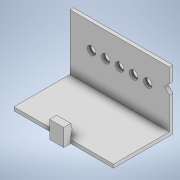
# Autodesk Inventor part: PCB_Case02B
Saved by Autodesk Inventor 2021 (Build 250183000, 183)
## iProperties
Created: 2021-02-15
Part Number: PCB_Case02B
Material: Generic
Document SubType Name: Modeling
Designer: Ryan
Density: 1 g/cm^3
Appearance: Default
Author: Ryan
Autodesk Inventor part; units mm, degrees
ref_plane "YZ Plane" through (0, 0, 0) normal (1, 0, 0) x (0, 1, 0)
ref_plane "XZ Plane" through (0, 0, 0) normal (0, 1, 0) x (-1, 0, 0)
ref_plane "XY Plane" through (0, 0, 0) normal (0, 0, 1) x (1, 0, 0)
sketch "Sketch1" plane through (0, 0, 0) normal (0, 1, 0) x (-1, 0, 0)
  line L0 (45.085, 26.9875) -> (-45.085, 26.9875)
  line L1 (-45.085, 26.9875) -> (-45.085, -26.9875)
  line L2 (-45.085, -26.9875) -> (45.085, -26.9875)
  line L3 (45.085, -26.9875) -> (45.085, 26.9875)
  point P0 (0, 0)
  dimension "d0" = 90.17
  dimension "d1" = 45.085
  dimension "d2" = 53.975
  dimension "d3" = 26.9875
  constraints: 8 end point, 2 parallel, 1 horizontal, 1 perpendicular
  measures "d0" distance of L0.start L0.end
  measures "d1" distance from line of point (0, 0) L3
  measures "d2" distance of L2.end L0.start
  measures "d3" distance from line of point (0, 0) L0
extrude "Extrusion1" add sketch "Sketch1" along normal blind 53.975
sketch "Sketch2" plane through (45.085, 0, 26.9875) normal (1, 0, 0) x (0, 0, -1)
  line L0 (0, 53.975) -> (53.975, 53.975) projected
  line L1 (0, 53.975) -> (50.8, 53.975)
  line L2 (50.8, 53.975) -> (50.8, 3.175)
  line L3 (50.8, 3.175) -> (0, 3.175)
  line L4 (0, 3.175) -> (0, 53.975)
  line L5 (0, 0) -> (53.975, 0) projected
  line L6 (53.975, 0) -> (53.975, 53.975) projected
  point P0 (26.9875, 0)
  dimension "d6" = 3.175
  dimension "d7" = 3.175
  constraints: 8 end point, 2 parallel, 1 horizontal, 1 perpendicular
  measures "d6" distance between parallel lines of L5 L3
  measures "d7" distance between parallel lines of L6 L2
extrude "Extrusion2" cut sketch "Sketch2" against normal through all
sketch "Sketch3" plane through (0, 0, 0) normal (0, -1, 0) x (1, 0, 0)
  line L0 (-6.35, 23.8125) -> (6.35, 23.8125)
  line L1 (6.35, 23.8125) -> (6.35, 33.3375)
  line L2 (6.35, 33.3375) -> (-6.35, 33.3375)
  line L3 (-6.35, 33.3375) -> (-6.35, 23.8125)
  line L4 (1.9102, 23.8125) -> (1.9102, 26.9875) construction
  line L5 (-45.085, 26.9875) -> (45.085, 26.9875) projected
  point P0 (0, 0)
  dimension "d10" = 12.7
  dimension "d11" = 9.525
  dimension "d12" = 3.175
  dimension "d13" = 6.35
  constraints: 10 end point, 2 parallel, 2 point on line, 1 horizontal, 1 perpendicular, 1 vertical
  measures "d10" distance of L1.end L2.end
  measures "d11" distance of L0.end L1.end
  measures "d12" distance of L4.start L4.end
  measures "d13" distance from line of point (0, 0) L3
extrude "Extrusion3" add sketch "Sketch3" against normal blind 15.875
sketch "Sketch4" plane through (6.35, 0, 33.3375) normal (1, 0, 0) x (0, 0, -1)
  line L0 (9.525, 3.175) -> (6.35, 3.175) projected
  line L1 (9.525, 3.175) -> (9.525, 15.875) projected
  line L2 (0, 15.875) -> (9.525, 15.875) projected
  line L3 (6.35, 0) -> (6.35, 3.175) projected
  line L4 (6.35, 3.175) -> (6.35, 5.715)
  line L5 (6.35, 5.715) -> (6.35, 15.875) construction
  line L6 (6.35, 5.715) -> (7.62, 10.795)
  line L7 (7.62, 10.795) -> (6.35, 15.875)
  point P0 (33.3375, 0)
  dimension "d19" = 1.27
  dimension "d20" = 10.16
  constraints: 8 end point, 2 point on line, 1 equal length, 1 vertical
  measures "d19" distance from line of L5 L6.end
  measures "d20" distance of L5.end L4.end
extrude "Extrusion4" cut sketch "Sketch4" against normal blind 15.875
sketch "Sketch5" plane through (45.085, 0, -26.9875) normal (0, 0, -1) x (-1, 0, 0)
  line L0 (19.6342, 31.75) -> (32.3596, 31.75) construction
  line L1 (32.3596, 31.75) -> (45.085, 31.75) construction
  line L2 (45.085, 31.75) -> (57.8104, 31.75) construction
  line L3 (57.8104, 31.75) -> (70.5358, 31.75) construction
  circle A0 centre (19.6342, 31.75) radius 3.81
  circle A1 centre (32.3596, 31.75) radius 3.81
  circle A2 centre (45.085, 31.75) radius 3.81
  circle A3 centre (57.8104, 31.75) radius 3.81
  circle A4 centre (70.5358, 31.75) radius 3.81
  line L4 (19.6342, 31.75) -> (5.2747, 31.75) construction
  line L5 (70.5358, 31.75) -> (84.8953, 31.75) construction
  line L6 (0, 53.975) -> (90.17, 53.975) projected
  point P0 (45.085, 0)
  point P1 (86.995, 3.175)
  point P2 (3.175, 3.175)
  dimension "d23" = 12.7254
  dimension "d24" = 7.62
  dimension "d26" = 22.225
  constraints: 12 end point, 6 collinear, 5 centre point, 5 coincident, 4 equal radius, 3 point on line
  measures "d23" distance of L0.start L0.end
  measures "d24" diameter of A0
  measures "d26" distance between parallel lines of L6 L5
extrude "Extrusion5" cut sketch "Sketch5" against normal blind 15.875
sketch "Sketch6" plane through (45.085, 3.175, -23.8125) normal (0, 0, 1) x (1, 0, 0)
  line L0 (0, 37.8968) -> (-4.572, 33.3248)
  line L1 (-4.572, 33.3248) -> (0, 28.7528)
  line L2 (0, 50.8) -> (-90.17, 50.8) projected
  line L3 (0, 37.8968) -> (0, 50.8)
  line L4 (0, 28.7528) -> (0, 25.3386)
  line L5 (0, 50.8) -> (0, 0) projected
  point P0 (-45.085, -3.175)
  dimension "d31" = 12.9032
  dimension "d32" = 45
  dimension "d33" = 45
  dimension "d35" = 4.572
  constraints: 8 end point, 1 perpendicular, 1 vertical
  measures "d31" distance from line of L2 L0.start
  measures "d32" angle of L5 L0
  measures "d33" angle of L4 L1
  measures "d35" distance from line of L5 L0.end
extrude "Extrusion6" cut sketch "Sketch6" against normal blind 25.4
equation "\"d1\" = 0.5 * d0"
equation "\"d3\" = 0.5 * d2"
equation "\"d13\" = 0.5 * d10"
body "Solid1"
